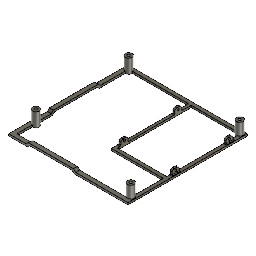
Mobo+HDD (Autodesk Fusion 360 design; units mm, degrees)
Autodesk Fusion 360 part; units mm, degrees
sketch "Sketch4" plane through (0, 0, 0) normal (0, 0, 1) x (1, 0, 0)
  line L0 (0, 0) -> (170, 0)
  line L1 (170, 0) -> (170, 170)
  line L2 (170, 170) -> (0, 170)
  line L3 (0, 170) -> (0, 0)
  line L4 (165, 6) -> (165, 165)
  line L5 (165, 165) -> (6, 165)
  line L6 (6, 165) -> (6, 6)
  line L7 (6, 6) -> (165, 6)
  circle A0 centre (6, 33) radius 2
  circle A1 centre (6, 33) radius 5
  circle A2 centre (6, 165) radius 2
  circle A3 centre (6, 165) radius 5
  circle A4 centre (164, 10) radius 2
  circle A5 centre (164, 10) radius 5
  line L8 (165, 165) -> (95, 165)
  line L9 (95, 165) -> (95, 60)
  line L10 (95, 60) -> (165, 60)
  line L11 (165, 60) -> (165, 165)
  line L12 (91, 165) -> (91, 55)
  line L13 (91, 55) -> (165, 55)
  line L14 (0, 55) -> (6, 55)
  line L15 (0, 60) -> (6, 60)
  line L16 (0, 120) -> (6, 120)
  line L17 (0, 125) -> (6, 125)
  line L18 (25.3171, 6) -> (25.3171, 0)
  line L19 (30.3171, 6) -> (30.3171, 0)
  line L20 (90.3171, 6) -> (90.3171, 0)
  line L21 (95.3171, 6) -> (95.3171, 0)
  line L22 (92, 75) -> (95, 75)
  line L23 (95, 75) -> (95, 65)
  line L24 (95, 65) -> (92, 65)
  line L25 (92, 65) -> (92, 75)
  line L26 (165, 65) -> (168, 65)
  line L27 (168, 65) -> (168, 75)
  line L28 (168, 75) -> (165, 75)
  line L29 (165, 75) -> (165, 65)
  line L30 (95, 151.5) -> (92, 151.5)
  line L31 (92, 151.5) -> (92, 141.5)
  line L32 (92, 141.5) -> (95, 141.5)
  line L33 (95, 141.5) -> (95, 151.5)
  line L34 (165, 151.5) -> (168, 151.5)
  line L35 (168, 151.5) -> (168, 141.5)
  line L36 (168, 141.5) -> (165, 141.5)
  line L37 (165, 141.5) -> (165, 151.5)
  circle A6 centre (164, 165) radius 2
  circle A7 centre (164, 165) radius 5
  point P0 (6, 33)
  point P1 (164, 10)
  point P2 (164, 165)
  dimension "d44" = 170
  dimension "d45" = 170
  dimension "d47" = 33
  dimension "d48" = 10
  dimension "d49" = 4
  dimension "d50" = 10
  dimension "d51" = 4
  dimension "d52" = 10
  dimension "d55" = 4
  dimension "d56" = 10
  dimension "d57" = 70
  dimension "d58" = 105
  dimension "d60" = 60
  dimension "d61" = 5
  dimension "d63" = 5
  dimension "d64" = 5
  dimension "d65" = 5
  dimension "d66" = 60
  dimension "d67" = 105
  dimension "d75" = 5
  dimension "d76" = 6
  dimension "d77" = 6
  dimension "d78" = 5
  dimension "d79" = 6
  dimension "d80" = 4
  dimension "d81" = 3
  dimension "d82" = 10
  dimension "d83" = 10
  dimension "d84" = 3
  dimension "d85" = 10
  dimension "d86" = 3
  dimension "d87" = 3
  dimension "d88" = 10
  dimension "d89" = 13.5
  dimension "d90" = 13.5
  dimension "d91" = 66.5
  dimension "d92" = 66.5
  dimension "d93" = 6
  dimension "d94" = 4
  dimension "d95" = 10
  constraint horizontal L0
  constraint vertical L1
  constraint horizontal L2
  constraint vertical L3
  constraint coincident L0.start L3.end
  constraint coincident L6 P0
  constraint coincident P0 A0.centre
  constraint coincident L5.end L6.start
  constraint concentric A2 A3
  constraint coincident P1 A4.centre
  constraint horizontal L8
  constraint vertical L9
  constraint horizontal L10
  constraint vertical L11
  constraint parallel L9 L12
  constraint parallel L10 L13
  constraint coincident L5 L12.start
  constraint coincident L4 L13.end
  constraint coincident L3 L14.start
  constraint coincident L6 L14.end
  constraint perpendicular L6 L14
  constraint coincident L3 L15.start
  constraint coincident L6 L15.end
  constraint perpendicular L6 L15
  constraint coincident L3 L16.start
  constraint coincident L6 L16.end
  constraint perpendicular L6 L16
  constraint coincident L3 L17.start
  constraint coincident L6 L17.end
  constraint perpendicular L6 L17
  constraint coincident L7 L18.start
  constraint coincident L0 L18.end
  constraint perpendicular L0 L18
  constraint coincident L7 L19.start
  constraint coincident L0 L19.end
  constraint perpendicular L0 L19
  constraint coincident L7 L21.start
  constraint coincident L0 L21.end
  constraint perpendicular L0 L21
  constraint coincident L0 L20.end
  constraint coincident L7 L20.start
  constraint parallel L1 L4
  constraint parallel L2 L5
  constraint parallel L3 L6
  constraint parallel L0 L7
  constraint horizontal L22
  constraint vertical L23
  constraint horizontal L24
  constraint vertical L25
  constraint coincident L9 L23.end
  constraint horizontal L26
  constraint vertical L27
  constraint horizontal L28
  constraint vertical L29
  constraint coincident L4 L26.start
  constraint horizontal L30
  constraint vertical L31
  constraint horizontal L32
  constraint vertical L33
  constraint coincident L9 L30.start
  constraint horizontal L34
  constraint vertical L35
  constraint horizontal L36
  constraint vertical L37
  constraint coincident L11 L34.start
  constraint coincident L5 P2
  constraint coincident L8 P2
  constraint coincident P2 A6.centre
  measures "d44" distance of L0.start L2.end
  measures "d45" distance of L0.start L0.end
  measures "d47" distance of L0 P0
  measures "d48" distance of L0 P1
  measures "d49" diameter of A0
  measures "d50" diameter of A1
  measures "d51" diameter of A2
  measures "d52" diameter of A3
  measures "d55" diameter of A4
  measures "d56" diameter of A5
  measures "d57" distance of L4.end L8.end
  measures "d58" distance of L4.end L10.end
  measures "d60" distance of L15 L16
  measures "d61" distance of L16 L17
  measures "d63" distance of L14 L15
  measures "d64" distance of L18 L19
  measures "d65" distance of L20 L21
  measures "d66" distance of L19 L20
  measures "d67" distance of L5.end L15
  measures "d75" distance of L2 L5
  measures "d76" distance of L3 L6
  measures "d77" distance of L0 L7
  measures "d78" distance of L1 L4
  measures "d79" distance of L1 P1
  measures "d80" distance of L9 L12
  measures "d81" distance of L22.start L22.end
  measures "d82" distance of L22.start L24.end
  measures "d83" distance of L26.start L28.end
  measures "d84" distance of L26.start L26.end
  measures "d85" distance of L30.start L32.end
  measures "d86" distance of L30.start L30.end
  measures "d87" distance of L34.start L34.end
  measures "d88" distance of L34.start L36.end
  measures "d89" distance of L5 L30
  measures "d90" distance of L8 L34
  measures "d91" distance of L22.start L31.end
  measures "d92" distance of L27.end L35.end
  measures "d93" distance of L1 P2
  measures "d94" diameter of A6
  measures "d95" diameter of A7
extrude "Extrude8" add sketch "Sketch4" along normal blind 3 contours L0 L3 L6 L7 A1 L14 L18 | L0 L7 L18 L19 | L3 L6 L14 L15 | L0 L7 L20 L21 | L3 L6 L16 L17 | L0 L1 L2 L4 L7 A5 L11 L21 L26 L27 L28 L34 L35 L36 A7 | L2 L3 L6 A3 L17 | L2 L5 A3 L8 A7 | L4 L5 L8 L11 A6 A7 | L4 L5 L9 L10 L12 L13 L22 L24 L25 L30 L31 L32 | L4 L5 L8 L11 A6 | L4 L11 L34 L35 L36 L37 | L9 L30 L31 L32 L33 | L4 L11 L26 L27 L28 L29 | L9 L22 L23 L24 L25 picked at (164.287, 168.9812) picked at (163.0074, 165.0994) makes body 2 at (113.8781, 4, 0) makes body 2 at (3.7516, 133.3519, 0) makes body 1 at (12.1057, 2, 0)
extrude "Extrude9" add sketch "Sketch4" along normal blind 20 contours L6 A0 A1 | L6 A0 A1 | L4 L7 A4 A5 | L4 L7 A4 A5 | L5 L6 A2 A3 | L5 L6 A2 A3 | L4 L5 L8 L11 A6 A7 | L4 L5 L8 L11 A6 A7 bodies 2 1
extrude "Extrude10" add sketch "Sketch4" along normal blind 3 from surface at 3 contours L0 L7 L18 L19 | L3 L6 L14 L15 | L0 L7 L19 L20 | L3 L6 L15 L16 | L0 L7 L20 L21 | L3 L6 L16 L17 bodies 2 1
extrude "Extrude11" add sketch "Sketch4" along normal blind 10 contours L4 L11 L34 L35 L36 L37 | L9 L30 L31 L32 L33 | L4 L11 L26 L27 L28 L29 | L9 L22 L23 L24 L25 bodies 2
sketch "Sketch5" plane through (168, 0, 0) normal (1, 0, 0) x (0, 1, 0)
  line L0 (141.5, 3) -> (151.5, 3)
  line L1 (151.5, 3) -> (151.5, 10)
  line L2 (151.5, 10) -> (141.5, 10)
  line L3 (141.5, 10) -> (141.5, 3)
  circle A0 centre (146.5, 7) radius 1.5
  line L4 (65, 3) -> (75, 3)
  line L5 (75, 3) -> (75, 10)
  line L6 (75, 10) -> (65, 10)
  line L7 (65, 10) -> (65, 3)
  circle A1 centre (70, 7) radius 1.5
  dimension "d98" = 3
  dimension "d99" = 3
  dimension "d100" = 5
  dimension "d101" = 3
  dimension "d102" = 3
  measures "d98" diameter of A0
  measures "d99" distance of L2 A0.centre
  measures "d100" distance of L1 A0.centre
  measures "d101" diameter of A1
  measures "d102" distance of L6 A1.centre
extrude "Extrude12" cut sketch "Sketch5" against normal blind 80 contours A0 | A1 bodies 2
chamfer "Chamfer2" distance 3 angle 45 8 edges at (3, 125, 6) (3, 55, 6) (25.3171, 3, 6) (95.3171, 3, 6) (3, 120, 0) (3, 60, 0) (30.3171, 3, 0) (90.3171, 3, 0) on bodies 2
fillet "Fillet1" radius 1 12 edges at (93.5, 75, 3) (93.5, 65, 3) (92, 70, 3) (93.5, 141.5, 3) (93.5, 151.5, 3) (92, 146.5, 3) (166.5, 151.5, 3) (168, 146.5, 3) (166.5, 141.5, 3) (166.5, 75, 3) (168, 70, 3) (166.5, 65, 3) on bodies 2
fillet "Fillet1" radius 3 8 edges at (93.5, 65, 10) (93.5, 75, 10) (93.5, 141.5, 10) (93.5, 151.5, 10) (166.5, 151.5, 10) (166.5, 141.5, 10) (166.5, 75, 10) (166.5, 65, 10) on bodies 2
named bodies: "Mini-ITX"
